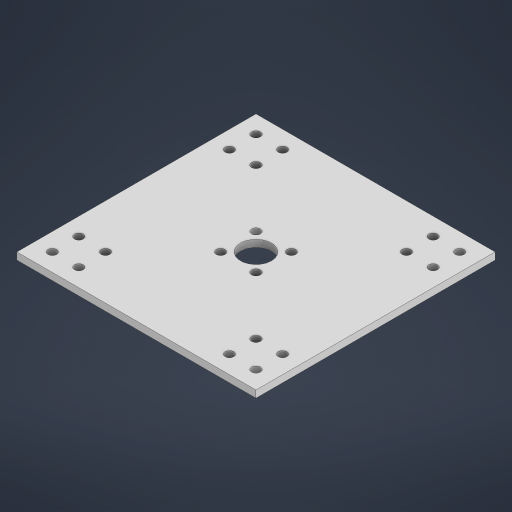
# Autodesk Inventor part: TurretMotorTopPlate
Saved by Autodesk Inventor 2024 (Build 280153000, 153)
## iProperties
Created: 2023-10-20
Part Number: TurretMotorTopPlate
Material: Generic
Document SubType Name: Modeling
Designer: avsar
Density: 1 g/cm^3
Appearance: Default
Author: avsar
Autodesk Inventor part; units mm, degrees
ref_plane "YZ Plane" through (0, 0, 0) normal (1, 0, 0) x (0, 1, 0)
ref_plane "XZ Plane" through (0, 0, 0) normal (0, 1, 0) x (-1, 0, 0)
ref_plane "XY Plane" through (0, 0, 0) normal (0, 0, 1) x (1, 0, 0)
sketch "Sketch1" plane through (0, 0, 0) normal (0, 1, 0) x (-1, 0, 0)
  line L0 (54, 54) -> (-54, 54)
  line L1 (-54, 54) -> (-54, -54)
  line L2 (-54, -54) -> (54, -54)
  line L3 (54, -54) -> (54, 54)
  line L4 (54, 54) -> (-54, -54) construction
  line L5 (-54, 54) -> (54, -54) construction
  point P0 (0, 0)
  dimension "d0" = 108
  dimension "d1" = 108
  constraints: 12 end point, 2 midpoint, 2 parallel, 1 horizontal, 1 perpendicular
  measures "d0" distance of L2.end L1.end
  measures "d1" distance of L1.end L0.end
extrude "Extrusion1" add sketch "Sketch1" along normal mid plane 3.175
sketch "Sketch2" plane through (0, 1.5875, 0) normal (0, 1, 0) x (1, 0, 0)
  circle A0 centre (-40, -40) radius 2.5 construction
  circle A1 centre (-46, -46) radius 2
  circle A2 centre (-34, -46) radius 2
  circle A3 centre (-34, -34) radius 2
  circle A4 centre (-46, -34) radius 2
  circle A5 centre (34, -46) radius 2
  circle A6 centre (34, -34) radius 2
  circle A7 centre (46, -34) radius 2
  circle A8 centre (46, -46) radius 2
  circle A9 centre (46, 34) radius 2
  circle A10 centre (34, 34) radius 2
  circle A11 centre (34, 46) radius 2
  circle A12 centre (46, 46) radius 2
  circle A13 centre (-34, 46) radius 2
  circle A14 centre (-34, 34) radius 2
  circle A15 centre (-46, 34) radius 2
  circle A16 centre (-46, 46) radius 2
  point P0 (0, 0)
  dimension "d4" = 5
  dimension "d5" = 40
  dimension "d6" = 40
  dimension "d7" = 4
  dimension "d8" = 6
  dimension "d9" = 6
  dimension "d12" = 360
  dimension "d16" = 360
  constraints: 17 centre point, 42 other
  measures "d4" diameter of A0
  measures "d5" horizontal distance of point (0, 0) A0.centre
  measures "d6" horizontal distance of point (0, 0) A0.centre
  measures "d7" diameter of A1
  measures "d8" horizontal distance of A0.centre A1.centre
  measures "d9" horizontal distance of A0.centre A1.centre
extrude "Extrusion2" cut sketch "Sketch2" against normal through all
sketch "Sketch3" plane through (0, 1.5875, 0) normal (0, 1, 0) x (1, 0, 0)
  circle A0 centre (0, 0) radius 7
  circle A1 centre (-8, 8) radius 2
  circle A2 centre (-8, -8) radius 2
  circle A3 centre (8, -8) radius 2
  circle A4 centre (8, 8) radius 2
  dimension "d20" = 14
  dimension "d21" = 4
  dimension "d22" = 8
  dimension "d23" = 8
  dimension "d26" = 360
  constraints: 5 centre point, 1 coincident, 9 other
  measures "d20" diameter of A0
  measures "d21" diameter of A1
  measures "d22" horizontal distance of point (0, 0) A1.centre
  measures "d23" horizontal distance of point (0, 0) A1.centre
extrude "Extrusion3" cut sketch "Sketch3" against normal through all
body "Solid1"
